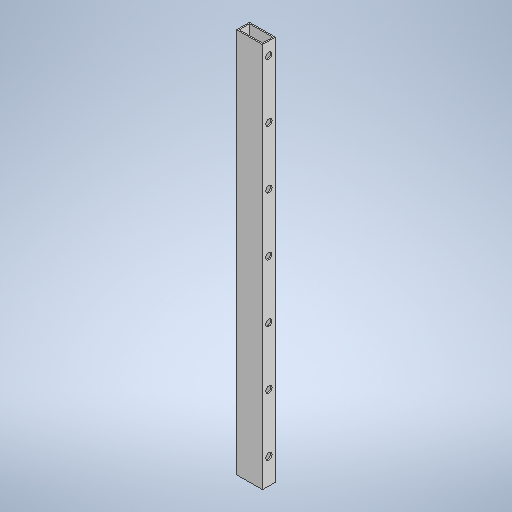
# Autodesk Inventor part: Wash way double
Saved by Autodesk Inventor 2025.4 (Build 294407000, 407)
## iProperties
Created: 2025-08-21
Part Number: Wash way double
Material: Generic
Document SubType Name: Modeling
Designer: pokla
Density: 1 g/cm^3
Appearance: Default
Author: pokla
Autodesk Inventor part; units mm, degrees
ref_plane "YZ Plane" through (0, 0, 0) normal (1, 0, 0) x (0, 1, 0)
ref_plane "XZ Plane" through (0, 0, 0) normal (0, 1, 0) x (-1, 0, 0)
ref_plane "XY Plane" through (0, 0, 0) normal (0, 0, 1) x (1, 0, 0)
sketch "Sketch1" plane through (0, 0, 0) normal (0, 0, 1) x (1, 0, 0)
  line L0 (-20, 10) -> (20, 10)
  line L1 (20, 10) -> (20, -10)
  line L2 (20, -10) -> (-20, -10)
  line L3 (-20, -10) -> (-20, 10)
  line L4 (-20, 10) -> (20, -10) construction
  line L5 (18, 8) -> (-18, 8)
  line L6 (-18, 8) -> (-18, -8)
  line L7 (-18, -8) -> (18, -8)
  line L8 (18, -8) -> (18, 8)
  point P0 (0, 0)
  point P1 (0, 0)
  dimension "d0" = 40
  dimension "d1" = 20
  dimension "d4" = 2
  constraints: 18 end point, 4 parallel, 2 perpendicular, 1 coincident, 1 horizontal, 1 midpoint, 3 other
  measures "d0" distance of L1.end L2.end
  measures "d1" distance of L2.end L0.start
  measures "d4" distance between parallel lines of L0 L5
extrude "Extrusion1" add sketch "Sketch1" along normal blind 600
sketch "Sketch2" plane through (0, 0, 0) normal (1, 0, 0) x (0, 1, 0)
  line L0 (-10, 0) -> (10, 0) projected
  line L1 (10, 0) -> (10, 600) construction
  line L2 (-10, 600) -> (10, 600) projected
  line L3 (-10, 0) -> (-10, 600) construction
  circle A0 centre (0, 580) radius 5
  point P0 (0, 0)
  point P1 (0, 600)
  dimension "d5" = 10
  dimension "d6" = 20
  constraints: 1 centre point, 1 midpoint, 1 vertical alignment
  measures "d5" diameter of A0
  measures "d6" distance from line of A0.centre L2
extrude "Extrusion2" cut sketch "Sketch2" along normal through all both and the other way through all
pattern_linear "Rectangular Pattern1" count 7 spacing 90 along (0, 0, -1) of "Extrusion2"
body "Solid1"
